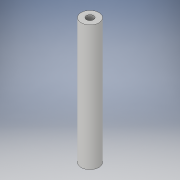
# Autodesk Inventor part: stem
Saved by Autodesk Inventor 2019 (Build 230136000, 136)
## iProperties
Created: 2020-02-19
Part Number: stem
Material: Generic
Document SubType Name: Modeling
Designer: FCI-L628
Density: 1 g/cm^3
Appearance: Default
Author: FCI-L628
Autodesk Inventor part; units mm, degrees
ref_plane "YZ Plane" through (0, 0, 0) normal (1, 0, 0) x (0, 1, 0)
ref_plane "XZ Plane" through (0, 0, 0) normal (0, 1, 0) x (-1, 0, 0)
ref_plane "XY Plane" through (0, 0, 0) normal (0, 0, 1) x (1, 0, 0)
sketch "Sketch1" plane through (0, 0, 0) normal (1, 0, 0) x (0, 1, 0)
  line L0 (12.1844, 23.3921) -> (-16.7086, 23.3921)
  line L1 (-16.7086, 23.3921) -> (-16.7086, 21.3356)
  line L2 (-16.7086, 21.3356) -> (12.1844, 21.3356)
  line L3 (12.1844, 21.3356) -> (12.1844, 23.3921)
  point P0 (0, 0)
  constraints: 8 end point, 2 parallel, 1 horizontal, 1 perpendicular
revolve "Revolution1" add sketch "Sketch1" angle 360 about axis through (0, 12.1844, 23.3921) along (0, -1, 0)
sketch "Sketch2" plane through (0, 12.1844, 23.3921) normal (0, 1, 0) x (1, 0, 0)
  circle A0 centre (0, 0) radius 0.8304
  point P0 (0, 23.3921)
  constraints: 1 centre point
extrude "Extrusion1" cut sketch "Sketch2" against normal blind 10
body "Solid1"
